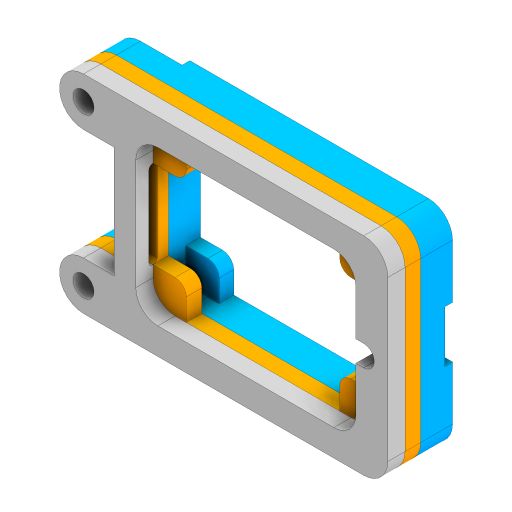
# Autodesk Inventor part: IMU Holder
Saved by Autodesk Inventor 2023 (Build 270158000, 158)
## iProperties
Created: 2022-07-03
Part Number: IMU Holder
Material: Generic
Document SubType Name: Modeling
Designer: Jochen Alt
Density: 1 g/cm^3
Appearance: Default
Author: Jochen Alt
Autodesk Inventor part; units mm, degrees
ref_plane "YZ Plane" through (0, 0, 0) normal (1, 0, 0) x (0, 1, 0)
ref_plane "XZ Plane" through (0, 0, 0) normal (0, 1, 0) x (-1, 0, 0)
ref_plane "XY Plane" through (0, 0, 0) normal (0, 0, 1) x (1, 0, 0)
sketch "Sketch1" plane through (0, 0, 0) normal (0, 0, 1) x (1, 0, 0)
  line L0 (-38.4722, 0) -> (38.4722, 0) construction
  line L1 (0, -24.3263) -> (0, 25.1372) construction
  line L2 (-27.4801, 0) -> (27.4801, 0) construction
  line L3 (0, -17.2601) -> (0, 18.071) construction
  line L4 (-16.256, 12.0396) -> (-12.4968, 12.0396)
  line L5 (19.05, 9.2456) -> (19.05, -9.2456)
  line L6 (16.256, -12.0396) -> (-12.4968, -12.0396)
  line L7 (-19.05, -9.2456) -> (-19.05, 9.2456) construction
  line L8 (-16.256, 9.2456) -> (-16.256, -9.2456) construction
  circle A0 centre (-16.256, 9.2456) radius 1.2192
  circle A1 centre (-16.256, -9.2456) radius 1.2192
  arc A2 (16.256, -1.2192) -> (16.256, 1.2192) centre (16.256, 0) ccw
  arc A3 (-16.256, 12.0396) -> (-19.05, 9.2456) centre (-16.256, 9.2456) ccw construction
  arc A4 (-19.05, -9.2456) -> (-16.256, -12.0396) centre (-16.256, -9.2456) ccw
  arc A5 (16.256, -12.0396) -> (19.05, -9.2456) centre (16.256, -9.2456) ccw
  arc A6 (19.05, 9.2456) -> (16.256, 12.0396) centre (16.256, 9.2456) ccw
  line L9 (-16.256, 9.2456) -> (-12.4968, 9.2456) construction
  line L10 (-12.4968, 6.4516) -> (-12.7, 6.4516)
  arc A7 (-16.256, 12.0396) -> (-16.256, 6.4516) centre (-16.256, 9.2456) ccw
  arc A8 (-12.4968, 6.4516) -> (-12.4968, 12.0396) centre (-12.4968, 9.2456) ccw
  line L11 (-16.256, -9.2456) -> (-12.4968, -9.2456) construction
  line L12 (-12.4968, -6.4516) -> (-16.256, -6.4516)
  arc A9 (-16.256, -6.4516) -> (-19.05, -9.2456) centre (-16.256, -9.2456) ccw
  arc A10 (-12.4968, -12.0396) -> (-12.4968, -6.4516) centre (-12.4968, -9.2456) ccw
  line L13 (-11.556, 9.2456) -> (-11.556, -9.2456) construction
  line L14 (-12.7, 6.4516) -> (-12.7, -6.4516)
  arc A11 (15.35, -2.643) -> (15.35, 2.643) centre (16.256, 0) ccw construction
  arc A12 (-12.4968, -6.4516) -> (-12.7, -6.459) centre (-12.4968, -9.2456) ccw
  line L15 (-12.4968, 12.0396) -> (16.256, 12.0396)
  line L16 (-12.4968, -12.0396) -> (-16.256, -12.0396)
  line L17 (-12.7, 6.4516) -> (-16.256, 6.4516)
  line L18 (-7.64, 8.965) -> (12.79, 8.965)
  line L19 (15.35, 6.405) -> (15.35, -6.405)
  line L20 (12.79, -8.965) -> (-7.64, -8.965)
  line L21 (-10.2, -6.405) -> (-10.2, 6.405)
  arc A13 (-7.64, 8.965) -> (-10.2, 6.405) centre (-7.64, 6.405) ccw
  arc A14 (15.35, 6.405) -> (12.79, 8.965) centre (12.79, 6.405) ccw
  arc A15 (12.79, -8.965) -> (15.35, -6.405) centre (12.79, -6.405) ccw
  arc A16 (-10.2, -6.405) -> (-7.64, -8.965) centre (-7.64, -6.405) ccw
  arc A17 (-6.335, -6.405) -> (-7.64, -5.1) centre (-7.64, -6.405) ccw
  arc A18 (12.77, -5.1) -> (11.465, -6.405) centre (12.77, -6.405) ccw
  arc A19 (11.465, 6.405) -> (12.77, 5.1) centre (12.77, 6.405) ccw
  arc A20 (-7.64, 5.1) -> (-6.335, 6.405) centre (-7.64, 6.405) ccw
  line L22 (-7.64, -5.1) -> (-10.2, -5.1)
  line L23 (-7.64, 5.1) -> (-10.2, 5.1)
  line L24 (-6.335, -6.405) -> (-6.335, -8.965)
  line L25 (11.465, -6.405) -> (11.465, -8.965)
  line L26 (12.77, -5.1) -> (15.35, -5.1)
  line L27 (12.77, 5.1) -> (15.35, 5.1)
  line L28 (11.465, 6.405) -> (11.465, 8.965)
  line L29 (-6.335, 6.405) -> (-6.335, 8.965)
  line L30 (16.256, -1.2192) -> (15.35, -1.2192)
  line L31 (16.256, 1.2192) -> (15.35, 1.2192)
  line L32 (16.256, 2.994) -> (19.05, 2.994)
  line L33 (16.256, -2.994) -> (19.05, -2.994)
  line L34 (-9.5028, -9.2456) -> (-9.5028, -12.0396)
  line L35 (-9.5028, 9.2456) -> (-9.5028, 12.0396)
  arc A21 (-12.7, 6.2585) -> (-11.4209, 12.0396) centre (-12.4968, 9.2456) ccw
  arc A22 (-11.4209, -12.0396) -> (-12.7, -6.2585) centre (-12.4968, -9.2456) ccw
  arc A23 (15.35, -2.8536) -> (16.256, -2.994) centre (16.256, 0) ccw
  line L36 (-10.2, 5.1) -> (-12.7, 5.1)
  line L37 (-10.2, -5.1) -> (-12.7, -5.1)
  arc A24 (16.256, 2.994) -> (15.35, 2.8536) centre (16.256, 0) ccw
  point P0 (-19.05, -9.2456)
  point P1 (-19.05, 9.2456)
  point P2 (0, 0)
  point P3 (19.05, -12.0396)
  point P4 (19.05, 12.0396)
  point P5 (-19.05, -12.0396)
  point P6 (-14.3764, 9.2456)
  point P7 (-14.3764, -9.2456)
  point P8 (-19.05, -9.2456)
  point P9 (-19.05, 9.2456)
  point P10 (0, 0)
  point P11 (-15.217, -8.6077)
  point P12 (-10.2, 8.965)
  point P13 (-10.2, -8.965)
  point P14 (19.05, 0)
  point P15 (15.0532, -0.1993)
  point P16 (15.0532, 0.1993)
  point P17 (-19.05, -9.2456)
  point P18 (-7.8539, 8.956)
  dimension "d9" = 38.1
  dimension "d10" = 24.0792
  dimension "d11" = 18.4912
  dimension "d12" = 2.4384
  dimension "d13" = 32.512
  dimension "d14" = 3.7592
  dimension "d15" = 4.7
  dimension "d16" = 6.35
  dimension "d20" = 17.93
  dimension "d21" = 25.55
  dimension "d22" = 2.56
  dimension "d33" = 10.2
  dimension "d34" = 0.2
  dimension "d40" = 17.8
  dimension "d41" = 10.2
  dimension "d42" = 0.2
  constraints: 74 end point, 49 point on circle, 46 tangent, 40 point on line, 24 centre point, 16 perpendicular, 13 equal radius, 9 parallel, 8 coincident, 7 horizontal, 3 midpoint, 2 vertical, 1 collinear, 1 concentric, 21 other
  measures "d9" distance of point (19.05, -12.04) point (-19.05, -12.04)
  measures "d10" distance of point (19.05, 12.04) point (19.05, -12.04)
  measures "d11" distance of L8.start L8.end
  measures "d12" diameter of A0
  measures "d13" distance from line of A2.centre L8
  measures "d14" distance of L9.end L8.start
  measures "d15" distance of L13.start L8.start
  measures "d16" distance between parallel lines of L14 L7
  measures "d20" distance of point (-10.2, -8.965) point (-10.2, 8.965)
  measures "d22" radius of A13
  measures "d33" distance between parallel lines of L3 L21
  measures "d34" radial gap between concentric circles of A22 A10
  measures "d40" distance between parallel lines of L28 L29
  measures "d41" distance between parallel lines of L22 L23
  measures "d42" radial gap between concentric circles of A8 A21
extrude "Extrusion1" add sketch "Sketch1" along normal blind 2.8 contours L4 A8 L10 L17 A7 | L15 A21 L14 L10 A8 | L15 L35 A21 | L15 A6 L5 L32 A24 L19 A14 L18 A13 L21 L36 L14 A21 L35 | L36 L21 L37 L14 | L37 L21 A16 L20 A15 L19 A23 L33 L5 A5 L6 L34 A22 L14 | L5 L33 A23 L19 L30 A2 L31 A24 L32 | A22 L6 A10 L12 L14 | L12 A10 L16 A4 A9 | L34 L6 A22
extrude "Extrusion2" add sketch "Sketch1" along normal blind 0.8 and the other way blind 0.9 contours L15 L35 A21 | L15 A6 L5 L32 A24 L19 A14 L18 A13 L21 L36 L14 A21 L35 | L36 L21 L37 L14 | L37 L21 A16 L20 A15 L19 A23 L33 L5 A5 L6 L34 A22 L14 | L21 A13 L18 L29 A20 L23 | A22 L6 A10 L12 L14 | L22 A17 L24 L20 A16 L21 | L34 L6 A22 | L27 A19 L28 L18 A14 L19
extrude "Extrusion3" add sketch "Sketch1" along normal blind 1.8 from surface at 2.8 separate body contours L4 A8 L10 L17 A7 | L15 A21 L14 L10 A8 | L15 L35 A21 | L15 A6 L5 L32 A24 L19 A14 L18 A13 L21 L36 L14 A21 L35 | L36 L21 L37 L14 | L37 L21 A16 L20 A15 L19 A23 L33 L5 A5 L6 L34 A22 L14 | L21 A13 L18 L29 A20 L23 | L5 L33 A23 L19 L30 A2 L31 A24 L32 | A22 L6 A10 L12 L14 | L22 A17 L24 L20 A16 L21 | L12 A10 L16 A4 A9 | L34 L6 A22 | L27 A19 L28 L18 A14 L19 | L19 A15 L20 L25 A18 L26
extrude "Extrusion4" add sketch "Sketch1" along normal blind 2 from surface at 4.6 separate body contours L4 A8 L10 L17 A7 | L15 A21 L14 L10 A8 | L15 L35 A21 | L15 A6 L5 L32 A24 L19 A14 L18 A13 L21 L36 L14 A21 L35 | L36 L21 L37 L14 | L37 L21 A16 L20 A15 L19 A23 L33 L5 A5 L6 L34 A22 L14 | L5 L33 A23 L19 L30 A2 L31 A24 L32 | A22 L6 A10 L12 L14 | L12 A10 L16 A4 A9 | L34 L6 A22
extrude "Extrusion5" cut sketch "Sketch1" along normal mid plane 1 from surface at 4.6 contours L36 L21 L37 L14 bodies 2 3
fillet "Fillet1" radius 0.5 4 edges at (-11.45, 5.1, 4.1) (-11.45, -5.1, 4.1) (-11.45, 5.1, 5.1) (-11.45, -5.1, 5.1)
